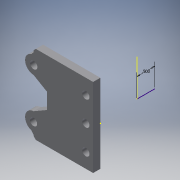
# Autodesk Inventor part: Hotend mount
Saved by Autodesk Inventor 2016 (Build 200138000, 138)
## iProperties
Created: 2016-06-02
Part Number: Hotend mount
Material: Generic
Document SubType Name: Modeling
Designer: Scott
Density: 1 g/cm^3
Appearance: Default
Author: Scott
Autodesk Inventor part; units mm, degrees
ref_plane "YZ Plane" through (0, 0, 0) normal (1, 0, 0) x (0, 1, 0)
ref_plane "XZ Plane" through (0, 0, 0) normal (0, 1, 0) x (-1, 0, 0)
ref_plane "XY Plane" through (0, 0, 0) normal (0, 0, 1) x (1, 0, 0)
sketch "Sketch1" plane through (0, 0, 0) normal (0, 0, 1) x (1, 0, 0)
  line L0 (-13.6843, -5.4848) -> (-23.1843, -10.9697) projected
  line L1 (-23.1843, -10.9697) -> (-32.6843, -5.4848) projected
  line L2 (-32.6843, -5.4848) -> (-32.6843, 5.4848) projected
  line L3 (-32.6843, 5.4848) -> (-23.1843, 10.9697) projected
  line L4 (-23.1843, 10.9697) -> (-13.6843, 5.4848) projected
  line L5 (-13.6843, 5.4848) -> (-13.6843, -5.4848) projected
  circle A0 centre (13.3507, 17.0193) radius 2.54 projected
  circle A1 centre (13.3507, -17.4028) radius 2.54 projected
  circle A2 centre (13.3507, 0) radius 2.54 projected
  circle A3 centre (-23.0489, 17.0193) radius 2.54 projected
  circle A4 centre (-23.2, -17.4028) radius 2.54 projected
  line L6 (-54.6393, -27.54) -> (18.4307, -27.54) projected
  line L7 (18.4307, -27.54) -> (18.4307, 27.54) projected
  line L8 (-54.6393, 27.54) -> (18.4307, 27.54) projected
  line L9 (-54.6393, -27.54) -> (-54.6393, 27.54) projected
  arc A5 (-23.1843, 23.0689) -> (-23.1843, 10.9697) centre (-23.0489, 17.0193) ccw
  line L10 (-23.1843, 10.9697) -> (-13.6843, 5.4848)
  line L11 (-13.6843, 5.4848) -> (-13.6843, -5.4848)
  line L12 (-13.6843, -5.4848) -> (-23.1843, -10.9697)
  line L13 (-23.1843, -23.6032) -> (-23.1843, -27.54)
  line L14 (-23.1843, 23.0689) -> (-23.1843, 27.54)
  line L15 (-23.1843, -27.54) -> (18.4307, -27.54)
  line L16 (18.4307, -27.54) -> (18.4307, 27.54)
  line L17 (18.4307, 27.54) -> (-23.1843, 27.54)
  arc A6 (-23.1843, -10.9697) -> (-23.1843, -23.6032) centre (-22.7708, -17.2864) ccw
  point P0 (0, 0)
  constraints: 16 end point, 5 collinear, 4 point on circle, 4 point on line, 2 centre point, 1 coincident, 1 horizontal, 1 perpendicular
extrude "Extrusion1" add sketch "Sketch1" along normal blind 5.08 contours L5 L4 A5 L14 L8 L7 L6 L13 A6 L0
chamfer "Chamfer1" distance 1.5875 angle 45 4 edges at (-23.1843, -27.54, 2.54) (-23.1843, 27.54, 2.54) (-23.1843, 23.0689, 2.54) (-23.1843, -23.6032, 2.54)
sketch "Sketch2" plane through (18.4307, -27.54, 0) normal (1, 0, 0) x (0, 0, -1)
  line L0 (25.4, 55.08) -> (25.4, 29.5535) projected
  line L1 (25.4, 29.5535) -> (38.1, 29.5535)
  point P0 (0, 27.54)
  dimension "d5" = 12.7
  constraints: 2 end point, 1 horizontal
  measures "d5" distance of L0.end L1.end
body "Solid1"
